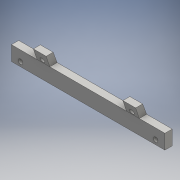
# Autodesk Inventor part: rpi_stabilizer
Saved by Autodesk Inventor 2016 (Build 200138000, 138)
## iProperties
Created: 2016-09-22
Part Number: rpi_stabilizer
Material: Generic
Document SubType Name: Modeling
Designer: Jakub
Density: 1 g/cm^3
Appearance: Default
Author: Jakub
Autodesk Inventor part; units mm, degrees
ref_plane "YZ Plane" through (0, 0, 0) normal (1, 0, 0) x (0, 1, 0)
ref_plane "XZ Plane" through (0, 0, 0) normal (0, 1, 0) x (-1, 0, 0)
ref_plane "XY Plane" through (0, 0, 0) normal (0, 0, 1) x (1, 0, 0)
sketch "Sketch1" plane through (0, 0, 0) normal (0, 1, 0) x (-1, 0, 0)
  line L0 (-42, 2.5) -> (42, 2.5)
  line L1 (42, 2.5) -> (42, -2.5)
  line L2 (42, -2.5) -> (-42, -2.5)
  line L3 (-42, -2.5) -> (-42, 2.5)
  line L4 (-42, 2.5) -> (42, -2.5) construction
  line L5 (42, 2.5) -> (-42, -2.5) construction
  point P0 (0, 0)
  dimension "d0" = 84
  dimension "d1" = 5
  constraints: 12 end point, 2 midpoint, 2 parallel, 1 horizontal, 1 perpendicular
  measures "d0" distance of L1.end L2.end
  measures "d1" distance of L0.end L1.end
extrude "Extrusion1" add sketch "Sketch1" along normal blind 4
sketch "Sketch2" plane through (0, 4, 0) normal (0, 1, 0) x (1, 0, 0)
  circle A0 centre (-37, 0) radius 1.25
  circle A1 centre (37, 0) radius 1.25
  line L0 (42, -2.5) -> (42, 2.5) projected
  line L1 (-42, -2.5) -> (-42, 2.5) projected
  point P0 (0, 0)
  dimension "d4" = 2.5
  dimension "d5" = 2.5
  dimension "d6" = 5
  dimension "d7" = 5
  constraints: 2 centre point
  measures "d4" diameter of A0
  measures "d5" diameter of A1
  measures "d6" distance from line of L0 A1.centre
  measures "d7" distance from line of L1 A0.centre
extrude "Extrusion2" cut sketch "Sketch2" against normal up to next
sketch "Sketch3" plane through (-42, 0, 2.5) normal (0, 0, 1) x (1, 0, 0)
  line L0 (84, 4) -> (0, 4) projected
  line L1 (0, 4) -> (84, 4)
  line L2 (84, 4) -> (84, 0)
  line L3 (84, 0) -> (0, 0)
  line L4 (0, 0) -> (0, 4)
  point P0 (42, 0)
  constraints: 8 end point, 2 parallel, 1 horizontal, 1 perpendicular
extrude "Extrusion3" add sketch "Sketch3" along normal blind 3
sketch "Sketch4" plane through (-42, 0, 5.5) normal (0, 0, 1) x (1, 0, 0)
  line L0 (84, 4) -> (70, 4)
  line L1 (84, 4) -> (0, 4) projected
  line L2 (0, 4) -> (14, 4)
  line L3 (14, 4) -> (21, 4)
  line L4 (21, 4) -> (21, -2)
  line L5 (21, -2) -> (14, -2)
  line L6 (14, -2) -> (14, 4)
  line L7 (70, 4) -> (63, 4)
  line L8 (63, 4) -> (63, -2)
  line L9 (63, -2) -> (70, -2)
  line L10 (70, -2) -> (70, 4)
  point P0 (42, 0)
  dimension "d12" = 14
  dimension "d13" = 14
  dimension "d14" = 7
  dimension "d15" = 6
  dimension "d16" = 7
  dimension "d17" = 6
  constraints: 20 end point, 4 parallel, 2 horizontal, 2 perpendicular, 2 point on line
  measures "d12" distance of L0.start L0.end
  measures "d13" distance of L1.end L2.end
  measures "d14" distance of L4.end L5.end
  measures "d15" distance of L3.end L4.end
  measures "d16" distance of L9.end L8.end
  measures "d17" distance of L8.end L7.end
extrude "Extrusion4" add sketch "Sketch4" along normal blind 6
sketch "Sketch5" plane through (28, -2, 5.5) normal (1, 0, 0) x (0, 0, -1)
  line L0 (0, 6) -> (-6, 3.8162)
  line L1 (-6, 0) -> (-6, 6) projected
  line L2 (0, 6) -> (6.3851, 6) construction
  line L3 (-6, 3.8162) -> (-6, 6)
  line L4 (0, 6) -> (-6, 6) projected
  line L5 (0, 6) -> (-6, 6)
  point P0 (5.5, 2)
  dimension "d20" = 160
  constraints: 8 end point, 2 horizontal, 1 collinear, 1 equal length, 1 point on line
  measures "d20" angle of L0 L2
extrude "Extrusion5" cut sketch "Sketch5" against normal through all
sketch "Sketch6" plane through (28, -2, 5.5) normal (1, 0, 0) x (0, 0, -1)
  line L0 (0, 0) -> (0, 2) projected
  line L1 (0, 0) -> (-6, 0) projected
  line L2 (0, 2) -> (-6, 0)
  point P0 (5.5, 2)
  constraints: 2 end point
extrude "Extrusion6" cut sketch "Sketch6" against normal through all
sketch "Sketch7" plane through (21, 1.8162, 11.5) normal (0, 0.9396926, 0.3420201) x (1, 0, 0)
  line L0 (0, -1.3052) -> (7, -1.3052) projected
  line L1 (3.5, -1.3052) -> (3.5, 3.1948)
  circle A0 centre (3.5, 3.1948) radius 1.25
  line L2 (-49, -1.3052) -> (-42, -1.3052) projected
  line L3 (-45.5, -1.3052) -> (-45.5, 3.1948)
  circle A1 centre (-45.5, 3.1948) radius 1.25
  point P0 (-21, 10.1853)
  dimension "d25" = 4.5
  dimension "d26" = 2.5
  dimension "d27" = 4.5
  dimension "d28" = 2.5
  constraints: 4 end point, 2 centre point, 2 coincident, 2 midpoint, 2 vertical
  measures "d25" distance of L1.start L1.end
  measures "d26" diameter of A0
  measures "d27" distance of L3.start L3.end
  measures "d28" diameter of A1
extrude "Extrusion7" cut sketch "Sketch7" against normal up to next
body "Solid1"
